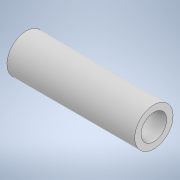
# Autodesk Inventor part: axle holder
Saved by Autodesk Inventor 2021 (Build 250183000, 183)
## iProperties
Created: 2021-02-20
Part Number: axle holder
Material: Generic
Document SubType Name: Modeling
Designer: bagal
Density: 1 g/cm^3
Appearance: Default
Author: bagal
Autodesk Inventor part; units mm, degrees
ref_plane "YZ Plane" through (0, 0, 0) normal (1, 0, 0) x (0, 1, 0)
ref_plane "XZ Plane" through (0, 0, 0) normal (0, 1, 0) x (-1, 0, 0)
ref_plane "XY Plane" through (0, 0, 0) normal (0, 0, 1) x (1, 0, 0)
sketch "Sketch1" plane through (0, 0, 0) normal (1, 0, 0) x (0, 1, 0)
  circle A0 centre (7.5231, 14.0593) radius 1.27
  circle A1 centre (7.5231, 14.0593) radius 1.905
  point P0 (0, 0)
  dimension "d0" = 2.54
  dimension "d1" = 3.81
  constraints: 2 centre point, 1 coincident
  measures "d0" diameter of A0
  measures "d1" diameter of A1
extrude "Extrusion1" add sketch "Sketch1" along normal blind 12.7
body "Solid1"
